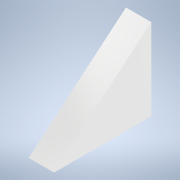
# Autodesk Inventor part: 40DegreeAngleTemplate
Saved by Autodesk Inventor 2020.2 (Build 242310000, 310)
## iProperties
Created: 2020-01-27
Part Number: 40DegreeAngleTemplate
Material: PET Plastic
Document SubType Name: Modeling
Designer: robst
Density: 1.541 g/cm^3
Appearance: Smooth - White
Author: robst
Autodesk Inventor part; units mm, degrees
ref_plane "YZ Plane" through (0, 0, 0) normal (1, 0, 0) x (0, 1, 0)
ref_plane "XZ Plane" through (0, 0, 0) normal (0, 1, 0) x (-1, 0, 0)
ref_plane "XY Plane" through (0, 0, 0) normal (0, 0, 1) x (1, 0, 0)
sketch "Sketch1" plane through (0, 0, 0) normal (1, 0, 0) x (0, 1, 0)
  line L0 (-103.1998, -115.9428) -> (-508.2392, 366.7644) projected
  line L1 (-482.8392, 336.4938) -> (-482.8392, 50.763) projected
  line L2 (-482.8392, 336.4938) -> (-401.2052, 239.2062)
  line L3 (-482.8392, 336.4938) -> (-482.8392, 239.2062)
  line L4 (-482.8392, 239.2062) -> (-401.2052, 239.2062)
  point P0 (0, 0)
  dimension "d0" = 127
  dimension "d1" = 40
  constraints: 6 end point, 2 point on line, 1 perpendicular
  measures "d0" distance of L2.end L1.start
  measures "d1" angle of L2 L1
extrude "Extrusion1" add sketch "Sketch1" against normal blind 25.4
sketch "Sketch3" plane through (0, 0, 0) normal (1, 0, 0) x (0, 0, -1)
  line L0 (-239.2062, -482.8392) -> (-336.4938, -482.8392) construction
  line L1 (-336.4938, -482.8392) -> (-239.2062, -447.4294) construction
  line L2 (-239.2062, -401.2052) -> (-239.2062, -482.8392) construction
  point P0 (0, 0)
  dimension "d4" = 20
  constraints: 2 end point, 1 point on line, 1 other
  measures "d4" angle of L1 L0
body "Solid1"
